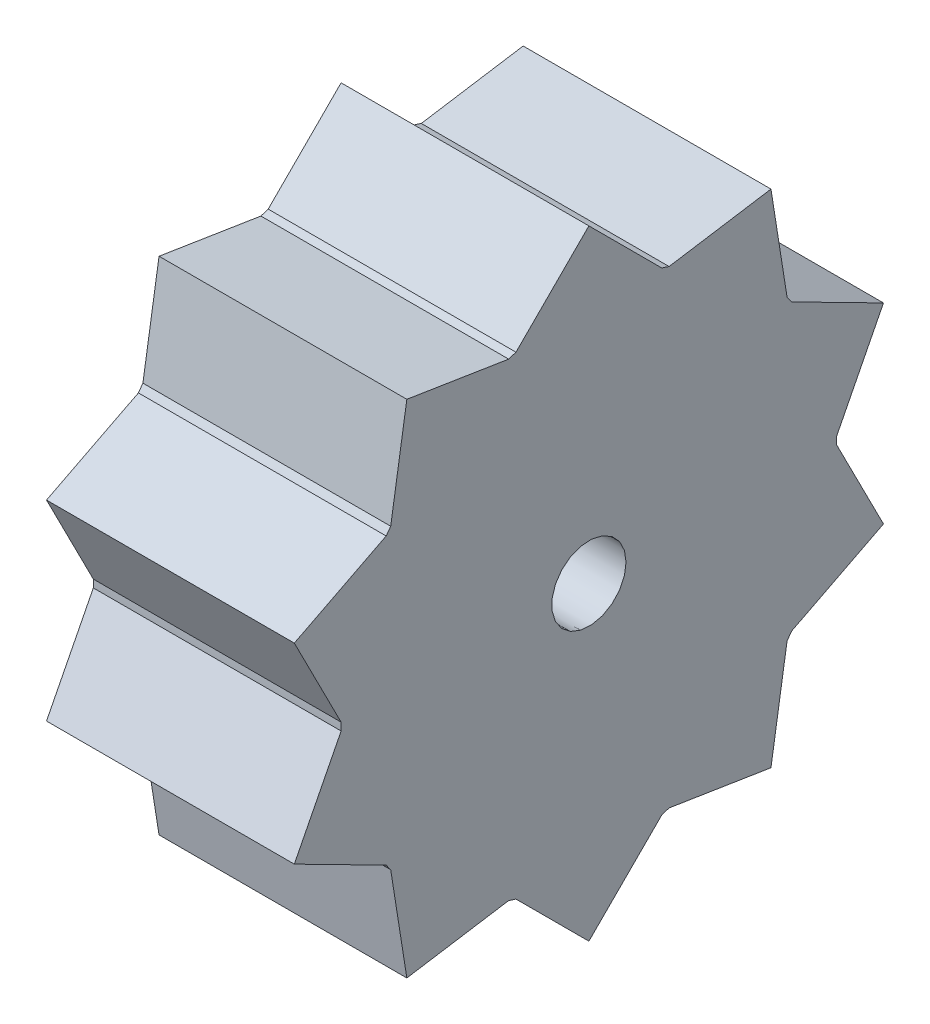
# Autodesk Inventor part: Finger Pinion
Saved by Autodesk Inventor 2023 (Build 270158000, 158)
## iProperties
Created: 2023-09-27
Part Number: Finger Pinion
Material: Generic
Document SubType Name: Modeling
Designer: Turnt
Density: 1 g/cm^3
Appearance: Default
Author: Turnt
Autodesk Inventor part; units mm, degrees
ref_plane "YZ Plane" through (0, 0, 0) normal (1, 0, 0) x (0, 1, 0)
ref_plane "XZ Plane" through (0, 0, 0) normal (0, 1, 0) x (-1, 0, 0)
ref_plane "XY Plane" through (0, 0, 0) normal (0, 0, 1) x (1, 0, 0)
sketch "Sketch1" plane through (0, 0, 0) normal (1, 0, 0) x (0, 1, 0)
  circle A0 centre (0, 0) radius 12.7
  arc A1 (12.1376, -3.7374) -> (12.1376, 3.7374) centre (0, 0) ccw
  dimension "d0" = 25.4
  constraints: 4 point on circle, 2 centre point, 1 coincident
  measures "d0" diameter of A0
extrude "Extrusion1" add sketch "Sketch1" along normal blind 12.7
sketch "Sketch2" plane through (12.7, 0, 0) normal (1, 0, 0) x (0, 0, -1)
  circle A0 centre (0, 0) radius 12.7 construction
  line L0 (0, 12.7) -> (3.175, 12.7) construction
  line L1 (0, 12.7) -> (-3.175, 12.7) construction
  line L2 (-3.175, 12.7) -> (0, 15.875) construction
  line L3 (0, 15.875) -> (3.175, 12.7) construction
  line L4 (0, 15.875) -> (-3.7374, 12.1376)
  line L5 (0, 15.875) -> (3.7374, 12.1376)
  arc A1 (3.7374, 12.1376) -> (-3.7374, 12.1376) centre (0, 0) ccw
  line L6 (-9.3311, 12.8431) -> (-10.1579, 7.6228)
  line L7 (-9.3311, 12.8431) -> (-4.1107, 12.0163)
  arc A2 (-4.1107, 12.0163) -> (-10.1579, 7.6228) centre (0, 0) ccw
  line L8 (-15.098, 4.9056) -> (-12.6985, 0.1963)
  line L9 (-15.098, 4.9056) -> (-10.3887, 7.3052)
  arc A3 (-10.3887, 7.3052) -> (-12.6985, 0.1963) centre (0, 0) ccw
  line L10 (-15.098, -4.9056) -> (-10.3887, -7.3052)
  line L11 (-15.098, -4.9056) -> (-12.6985, -0.1963)
  arc A4 (-12.6985, -0.1963) -> (-10.3887, -7.3052) centre (0, 0) ccw
  line L12 (-9.3311, -12.8431) -> (-4.1107, -12.0163)
  line L13 (-9.3311, -12.8431) -> (-10.1579, -7.6228)
  arc A5 (-10.1579, -7.6228) -> (-4.1107, -12.0163) centre (0, 0) ccw
  line L14 (0, -15.875) -> (3.7374, -12.1376)
  line L15 (0, -15.875) -> (-3.7374, -12.1376)
  arc A6 (-3.7374, -12.1376) -> (3.7374, -12.1376) centre (0, 0) ccw
  line L16 (9.3311, -12.8431) -> (10.1579, -7.6228)
  line L17 (9.3311, -12.8431) -> (4.1107, -12.0163)
  arc A7 (4.1107, -12.0163) -> (10.1579, -7.6228) centre (0, 0) ccw
  line L18 (15.098, -4.9056) -> (12.6985, -0.1963)
  line L19 (15.098, -4.9056) -> (10.3887, -7.3052)
  arc A8 (10.3887, -7.3052) -> (12.6985, -0.1963) centre (0, 0) ccw
  line L20 (15.098, 4.9056) -> (10.3887, 7.3052)
  line L21 (15.098, 4.9056) -> (12.6985, 0.1963)
  arc A9 (12.6985, 0.1963) -> (10.3887, 7.3052) centre (0, 0) ccw
  line L22 (9.3311, 12.8431) -> (4.1107, 12.0163)
  line L23 (9.3311, 12.8431) -> (10.1579, 7.6228)
  arc A10 (10.1579, 7.6228) -> (4.1107, 12.0163) centre (0, 0) ccw
  point P0 (-7.4649, 10.2745)
  point P1 (-12.0784, 3.9245)
  point P2 (-12.0784, -3.9245)
  point P3 (-7.4649, -10.2745)
  point P4 (0, -12.7)
  point P5 (7.4649, -10.2745)
  point P6 (12.0784, -3.9245)
  point P7 (12.0784, 3.9245)
  point P8 (7.4649, 10.2745)
  dimension "d6" = 3.175
  dimension "d7" = 3.175
  dimension "d8" = 45
  dimension "d11" = 360
  constraints: 48 end point, 33 point on circle, 10 centre point, 2 horizontal, 2 point on line, 2 tangent, 1 perpendicular, 81 other
  measures "d6" distance of L0.start L0.end
  measures "d7" distance of L0.start L1.end
  measures "d8" angle of L1 L2
extrude "Extrusion2" add sketch "Sketch2" against normal blind 12.7
sketch "Sketch3" plane through (12.7, 0, 0) normal (1, 0, 0) x (0, 0, -1)
  circle A0 centre (0, 0) radius 1.905
  dimension "d15" = 3.81
  constraints: 1 centre point, 1 coincident
  measures "d15" diameter of A0
extrude "Extrusion3" cut sketch "Sketch3" against normal blind 6.35
body "Solid1"
